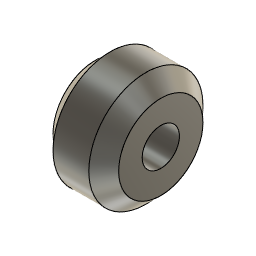
惰轮型号1 v1 (Autodesk Fusion 360 design; units mm, degrees)
Autodesk Fusion 360 part; units mm, degrees
sketch "草图1" plane through (0, 0, 0) normal (1, 0, 0) x (0, 1, 0)
  circle A0 centre (0, 0) radius 7.65
  circle A1 centre (0, 0) radius 2.5
  dimension "d1" = 15.3
  dimension "d2" = 5
  constraint coincident A0.centre A1.centre
  constraint concentric A0 A1
  measures "d1" diameter of A0
  measures "d2" diameter of A1
extrude "拉伸1" add sketch "草图1" along normal blind 8.8
chamfer "倒角1" distance 2 angle 45 2 edges at (0, -7.1323, -2.7664) (8.8, -7.1323, -2.7664)
